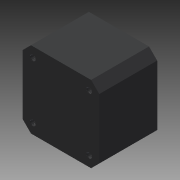
# Autodesk Inventor part: Top
Saved by Autodesk Inventor 2014 SP1 (Build 180222100, 222)
## iProperties
Created: 2017-07-08
Part Number: Top
Material: Типовые
Document SubType Name: Modeling
Designer: Stepan
Density: 1 g/cm^3
Appearance: Типовые
Author: Stepan
Autodesk Inventor part; units mm, degrees
ref_plane "YZ Plane" through (0, 0, 0) normal (1, 0, 0) x (0, 1, 0)
ref_plane "XZ Plane" through (0, 0, 0) normal (0, 1, 0) x (-1, 0, 0)
ref_plane "XY Plane" through (0, 0, 0) normal (0, 0, 1) x (1, 0, 0)
sketch "Эскиз1" plane through (0, 0, 0) normal (0, 1, 0) x (-1, 0, 0)
  line L0 (21.1, -21.1) -> (-21.1, -21.1)
  line L1 (-21.1, -21.1) -> (-21.1, 21.1)
  line L2 (-21.1, 21.1) -> (21.1, 21.1)
  line L3 (21.1, 21.1) -> (21.1, -21.1)
  line L4 (21.1, -21.1) -> (-21.1, 21.1) construction
  line L5 (-21.1, -21.1) -> (21.1, 21.1) construction
  line L6 (-15.55, 15.55) -> (15.55, 15.55) construction
  line L7 (15.55, 15.55) -> (15.55, -15.55) construction
  line L8 (15.55, -15.55) -> (-15.55, -15.55) construction
  line L9 (-15.55, -15.55) -> (-15.55, 15.55) construction
  line L10 (-15.55, 15.55) -> (15.55, -15.55) construction
  line L11 (15.55, 15.55) -> (-15.55, -15.55) construction
  circle A0 centre (-15.55, -15.55) radius 1.5
  circle A1 centre (15.55, -15.55) radius 1.5
  circle A2 centre (15.55, 15.55) radius 1.5
  circle A3 centre (-15.55, 15.55) radius 1.5
  point P0 (0, 0)
  dimension "d0" = 42.2
  dimension "d1" = 42.2
  dimension "d2" = 31.1
  dimension "d3" = 31.1
  dimension "d4" = 3
  dimension "d5" = 3
  dimension "d6" = 3
  dimension "d7" = 3
  constraints: 24 end point, 4 centre point, 4 coincident, 4 midpoint, 4 parallel, 2 horizontal, 2 perpendicular
  measures "d0" distance of L1.end L2.end
  measures "d1" distance of L0.end L1.end
  measures "d2" distance of L7.end L8.end
  measures "d3" distance of L6.end L7.end
  measures "d4" diameter of A0
  measures "d5" diameter of A1
  measures "d6" diameter of A2
  measures "d7" diameter of A3
extrude "Выдавливание1" add sketch "Эскиз1" along normal blind 32
chamfer "Фаска1" distance 4.5 angle 45 4 edges at (21.1, 16, -21.1) (21.1, 16, 21.1) (-21.1, 16, 21.1) (-21.1, 16, -21.1)
thread "Резьба1" size "M3x0.5" class "6H" standard "ANSI Metric M Profile" full length
thread "Резьба2" size "M3x0.5" class "6H" standard "ANSI Metric M Profile" full length
thread "Резьба3" size "M3x0.5" class "6H" standard "ANSI Metric M Profile" full length
thread "Резьба4" size "M3x0.5" class "6H" standard "ANSI Metric M Profile" full length
